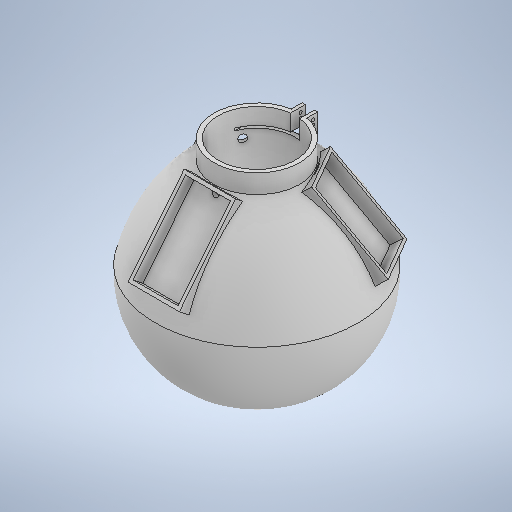
# Autodesk Inventor part: Water Sensor Bouy
Saved by Autodesk Inventor 2025 (Build 290162000, 162)
## iProperties
Created: 2024-06-17
Part Number: Water Sensor Bouy
Material: Generic
Document SubType Name: Modeling
Designer: track
Density: 1 g/cm^3
Appearance: Default
Mass: 1114.84 g
Surface Area: 2537.18 cm^2
Volume: 1114.84 cm^3
Author: track
## iProperties of the stored document Water Sensor Bouy_3DPrint.ipt
Created: 2024-06-17
Part Number: Water Sensor Bouy_3DPrint
Material: Generic
Document SubType Name: Modeling
Designer: track
Density: 1 g/cm^3
Appearance: Default
Author: track
Autodesk Inventor part; units mm, degrees
ref_plane "YZ Plane" through (0, 0, 0) normal (1, 0, 0) x (0, 1, 0)
ref_plane "XZ Plane" through (0, 0, 0) normal (0, 1, 0) x (-1, 0, 0)
ref_plane "XY Plane" through (0, 0, 0) normal (0, 0, 1) x (1, 0, 0)
sketch "Sketch1" plane through (0, 0, 0) normal (0, 0, 1) x (1, 0, 0)
  line L0 (0, 0) -> (0, 76.2)
  line L1 (31.2895, 0) -> (31.2895, 152.4)
  line L2 (31.2895, 76.2) -> (82.0895, 76.2)
  arc A0 (82.0895, 76.2) -> (31.2895, 152.4) centre (-41.8733, 48.5915) ccw
  arc A1 (31.2895, 0) -> (82.0895, 76.2) centre (6.0118, 71.8852) ccw
  line L3 (41.2895, 130.8894) -> (41.2895, 15.868)
  arc A2 (41.2895, 15.868) -> (72.1461, 74.8322) centre (6.0118, 71.8852) ccw
  arc A3 (72.1461, 74.8322) -> (41.2895, 130.8894) centre (-41.8733, 48.5915) ccw
  point P0 (31.2895, 50.8)
  dimension "d1" = 31.2895
  dimension "d3" = 0
  dimension "d74" = 152.4
  dimension "d75" = 50.8
  dimension "d76" = 76.2
  dimension "d78" = 127
  dimension "d83" = 10
  dimension "d128" = 83.1628
  dimension "d129" = 76.2
  constraints: 8 end point, 8 point on circle, 4 centre point, 2 vertical, 1 horizontal, 1 midpoint, 1 point on line, 2 other
  measures "d1" distance between parallel lines of L1 L0
  measures "d3" vertical distance of L0.start L1.start
  measures "d74" distance of L1.start L1.end
  measures "d75" distance of L2.start L2.end
  measures "d76" distance from line of L1.end L2
  measures "d78" radius of A0
  measures "d83" distance between parallel lines of L1 L3
  measures "d128" distance from line of L3 A0.centre
  measures "d129" radius of A1
revolve "Revolution1" add sketch "Sketch1" angle 360 about axis through (0, 0, 0) along (0, 1, 0) contours L1 L2 L3 A2 A3 A1 | L1 A0 L2 A3 L3
sketch "Sketch13" plane through (0, 0, 0) normal (0, 0, 1) x (1, 0, 0)
  line L0 (31.2895, 152.4) -> (-31.2895, 152.4) projected
  line L1 (0, 152.4) -> (0, 180.8136)
  line L2 (-31.2895, 152.4) -> (-31.2895, 165.1)
  line L3 (-31.2895, 165.1) -> (-33.8295, 165.1)
  line L4 (-33.8295, 165.1) -> (-33.8295, 150.5625)
  arc A0 (-31.2895, 152.4) -> (-82.0895, 76.2) centre (41.8733, 48.5915) ccw projected
  arc A1 (-31.2895, 152.4) -> (-33.8295, 150.5625) centre (41.8733, 48.5915) ccw
  point P0 (0, 0)
  dimension "d79" = 2.54
  dimension "d81" = 12.7
  constraints: 8 end point, 3 point on circle, 2 perpendicular, 2 vertical, 1 centre point, 1 concentric, 1 midpoint
  measures "d79" distance of L2.end L3.end
  measures "d81" distance of L0.end L2.end
revolve "Revolution2" add sketch "Sketch13" angle 260 about axis through (0, 152.4, 0) along (0, 1, 0) and the other way 90
sketch "Sketch17" plane through (0, 0, 0) normal (0, 0, 1) x (1, 0, 0)
  line L0 (0, 152.4) -> (0, 165.1) projected
  line L1 (0, 165.1) -> (-8.89, 165.1)
  line L2 (-8.89, 165.1) -> (-8.89, 150.5625)
  line L3 (-8.89, 150.5625) -> (0, 150.5625)
  line L4 (0, 150.5625) -> (0, 165.1)
  point P0 (0, 0)
  dimension "d91" = 8.89
  dimension "d92" = 14.5375
  constraints: 8 end point, 2 parallel, 1 horizontal, 1 perpendicular
  measures "d91" distance of L0.end L1.end
  measures "d92" distance of L1.end L2.end
extrude "Extrusion10" add sketch "Sketch17" along normal blind 2.54
sketch "Sketch18" plane through (0, 152.4, -31.2895) normal (1, 0, 0) x (0, 0, -1)
  line L0 (0, 12.7) -> (2.54, 12.7) projected
  line L1 (0, 0) -> (0, 12.7) projected
  arc A0 (2.54, -1.8375) -> (0, 0) centre (-73.1628, -103.8085) ccw projected
  line L2 (0, 0) -> (-0.4754, 0) projected
  arc A1 (50.8, -76.2) -> (0, 0) centre (-73.1628, -103.8085) ccw projected
  line L3 (0, 0) -> (2.54, -1.8375)
  line L4 (-31.2895, -1.8375) -> (2.54, -1.8375) projected
  line L5 (-33.8295, 12.7) -> (-33.8295, -1.8375) projected
  line L6 (8.89, -1.8375) -> (8.89, 12.7)
  line L7 (-33.8295, 12.7) -> (0, 12.7)
  line L8 (2.54, 12.7) -> (2.54, -1.8375) projected
  point P0 (-31.2895, -152.4)
  constraints: 6 end point, 1 perpendicular, 1 vertical
extrude "Extrusion11" add sketch "Sketch18" along normal blind 12.7 contours L0 L8 A0 L1
sketch "Sketch22" plane through (0, 0, 0) normal (1, 0, 0) x (0, 1, 0)
  arc A0 (150.5625, 33.8295) -> (76.2, 82.0895) centre (48.5915, -41.8733) ccw projected
  arc A1 (76.2, 82.0895) -> (0, 31.2895) centre (71.8852, 6.0118) ccw projected
  line L0 (128.1112, 57.15) -> (74.8322, 12.4436)
  line L1 (74.8322, -72.1461) -> (74.8322, 72.1461) projected
  line L2 (152.4, -31.2895) -> (165.1, -31.2895) projected
  line L3 (74.8322, 0) -> (165.1, 0)
  point P0 (0, 0)
  point P1 (74.8322, 0)
  point P2 (150.5625, 0)
  dimension "d125" = 50
  constraints: 4 end point, 1 horizontal, 1 midpoint, 1 point on circle, 1 point on line, 1 other
  measures "d125" angle of L1 L0
ref_plane "Work Plane6" through (0, 128.1112, 57.15) normal (0, 0.6261398, 0.7797108) x (-1, 0, 0)
sketch "Sketch23" plane through (0, 128.1112, 57.15) normal (0, 0.6261398, 0.7797108) x (-1, 0, 0)
  line L0 (18.25, -27.8894) -> (-18.25, -27.8894)
  line L1 (-18.25, -27.8894) -> (-18.25, 39.6106)
  line L2 (-18.25, 39.6106) -> (18.25, 39.6106)
  line L3 (18.25, 39.6106) -> (18.25, -27.8894)
  ellipse E0 centre (0, -53.2894) end of major axis (-33.8295, -53.2894) minor radius 21.182 (0, -74.4714) -> (-5.8744, -74.1496) ccw projected
  line L4 (-20.79, 42.1506) -> (-20.79, -30.4294)
  line L5 (-20.79, -30.4294) -> (20.79, -30.4294)
  line L6 (20.79, -30.4294) -> (20.79, 42.1506)
  line L7 (20.79, 42.1506) -> (-20.79, 42.1506)
  point P0 (0, 64.1058)
  point P1 (32.2678, -59.651)
  point P2 (33.734, -51.699)
  dimension "d130" = 36.5
  dimension "d131" = 67.5
  dimension "d132" = 25.4
  dimension "d133" = 18.25
  dimension "d134" = 2.54
  constraints: 16 end point, 4 parallel, 2 perpendicular, 1 horizontal, 4 other
  measures "d130" distance of L0.start L0.end
  measures "d131" distance of L0.end L1.end
  measures "d132" distance from line of point (0, -53.289) L0
  measures "d133" distance from line of point (0, -53.289) L1
  measures "d134" distance between parallel lines of L1 L4
extrude "Extrusion14" add sketch "Sketch23" against normal up to surface
sketch "Sketch24" plane through (0, 128.1112, 57.15) normal (0, 0.6261398, 0.7797108) x (-1, 0, 0)
  line L0 (18.25, -27.8894) -> (-18.25, -27.8894) projected
  line L1 (-18.25, -27.8894) -> (-18.25, 39.6106) projected
  line L2 (18.25, -27.8894) -> (-18.25, -27.8894)
  line L3 (-18.25, -27.8894) -> (-18.25, 39.6106)
  line L4 (-18.25, 39.6106) -> (18.25, 39.6106)
  line L5 (18.25, 39.6106) -> (18.25, -27.8894)
  point P0 (0, 64.1058)
  constraints: 8 end point, 2 parallel, 1 horizontal, 1 perpendicular
extrude "Extrusion15" cut sketch "Sketch24" against normal blind 10
sketch "Sketch25" plane through (0, 0, 0) normal (0, 0, 1) x (1, 0, 0)
  circle A0 centre (0, 143.5069) radius 3
  line L0 (-18.25, 149.8569) -> (18.25, 149.8569) projected
  line L1 (18.25, 149.8569) -> (18.25, 97.2264) projected
  point P0 (0, 0)
  dimension "d139" = 6
  dimension "d140" = 6.35
  dimension "d141" = 18.25
  constraints: 1 centre point
  measures "d139" diameter of A0
  measures "d140" distance from line of L0 A0.centre
  measures "d141" distance from line of L1 A0.centre
extrude "Extrusion16" cut sketch "Sketch25" along normal blind 63.5
sketch "Sketch26" plane through (0, 121.8498, 49.3529) normal (0, 0.6261398, 0.7797108) x (1, 0, 0)
  line L0 (-18.25, -39.6106) -> (-18.25, 27.8894) projected
  line L1 (18.25, 27.8894) -> (18.25, -39.6106) projected
  line L2 (-18.25, -14.2106) -> (18.25, -14.2106)
  line L3 (18.25, -14.2106) -> (18.25, -39.6106)
  line L4 (18.25, -39.6106) -> (-18.25, -39.6106)
  line L5 (-18.25, -39.6106) -> (-18.25, -14.2106)
  point P0 (0, -64.1058)
  point P1 (18.25, -14.2106)
  dimension "d144" = 25.4
  constraints: 8 end point, 2 parallel, 1 horizontal, 1 perpendicular, 1 point on line
  measures "d144" distance between parallel lines of L4 L2
extrude "Extrusion17" add sketch "Sketch26" against normal blind 10
pattern_circular "Circular Pattern4" count 3 over 360 about axis through (0, 157.8313, 0) along (0, 1, 0) of "Extrusion14", "Extrusion15", "Extrusion16", "Extrusion17"
sketch "Sketch27" plane through (0, 0, 0) normal (0, 1, 0) x (-1, 0, 0)
  line L0 (0, 0) -> (-82.0895, 0)
  circle A0 centre (0, 0) radius 82.0895 projected
  circle A1 centre (-50.8, 0) radius 3.175
  dimension "d150" = 6.35
  dimension "d151" = 50.8
  constraints: 2 end point, 1 centre point, 1 horizontal, 1 horizontal alignment, 1 point on line, 1 other
  measures "d150" diameter of A1
  measures "d151" distance of L0.start A1.centre
extrude "Extrusion18" cut sketch "Sketch27" along normal blind 33.02 contours A1 L0 | L0 A1
pattern_circular "Circular Pattern5" count 3 over 360 about axis through (0, 71.8852, 0) along (0, 1, 0) of "Extrusion18"
sketch "Sketch30" plane through (0, 165.1, -33.8295) normal (0, 1, 0) x (1, 0, 0)
  line L0 (0, -33.8295) -> (0, -36.3695) projected
  line L1 (12.7, 0) -> (12.7, -2.4744) projected
  circle A0 centre (0, -33.8295) radius 36.1348
  constraints: 1 coincident, 3 other
extrude "Extrusion20" cut sketch "Sketch30" against normal blind 15.24
sketch "Sketch31" plane through (0, 149.86, 0) normal (0, 1, 0) x (1, 0, 0)
  circle A0 centre (0, 0) radius 31.2895
  circle A1 centre (0, 0) radius 31.2895 projected
  circle A2 centre (0, 0) radius 34.7667 projected
  line L0 (6.35, 34.1819) -> (6.35, 43.0719)
  line L1 (6.35, 43.0719) -> (3.81, 43.0719)
  line L2 (3.81, 43.0719) -> (3.81, 34.5573)
  line L3 (-3.81, 34.5573) -> (-3.81, 43.0719)
  line L4 (-3.81, 43.0719) -> (-6.35, 43.0719)
  line L5 (-6.35, 43.0719) -> (-6.35, 34.1819)
  arc A3 (-6.35, 34.1819) -> (6.35, 34.1819) centre (0, 0) ccw
  line L6 (3.81, 34.5573) -> (3.81, 31.0567)
  line L7 (-3.81, 34.5573) -> (-3.81, 31.0567)
  dimension "d165" = 8.89
  dimension "d167" = 8.89
  dimension "d168" = 2.54
  dimension "d169" = 2.54
  dimension "d170" = 3.81
  constraints: 16 end point, 8 point on circle, 3 perpendicular, 2 centre point, 2 coincident, 2 parallel, 2 point on line, 2 vertical, 1 concentric
  measures "d165" distance of L0.start L0.end
  measures "d167" distance of L4.end L5.end
  measures "d168" distance of L3.end L4.end
  measures "d169" distance of L0.end L1.end
  measures "d170" distance from line of point (0, 0) L2
extrude "Extrusion21" add sketch "Sketch31" along normal blind 15.24 contours A0 L6 A2 L7 | L2 L1 L0 A2 | A2 L5 L4 L3 picked at (33.28, -2.7362)
sketch "Sketch32" plane through (-6.35, 149.86, -43.0719) normal (-1, 0, 0) x (0, 0, 1)
  line L0 (0, 15.24) -> (8.89, 15.24) projected
  line L1 (3.81, 15.24) -> (3.81, 0)
  line L2 (0, 0) -> (8.5146, 0) projected
  line L3 (0, 0) -> (0, 15.24) projected
  circle A0 centre (3.81, 11.43) radius 1.27
  circle A1 centre (3.81, 7.62) radius 1.27
  circle A2 centre (3.81, 3.81) radius 1.27
  point P0 (43.0719, -149.86)
  dimension "d173" = 3.81
  dimension "d174" = 2.54
  dimension "d175" = 7.62
  dimension "d176" = 3.81
  dimension "d177" = 3.81
  constraints: 4 point on line, 3 centre point, 2 end point, 2 equal radius, 1 midpoint, 1 vertical
  measures "d173" distance between parallel lines of L3 L1
  measures "d174" diameter of A1
  measures "d175" distance from line of L0 A1.centre
  measures "d176" distance of A1.centre A0.centre
  measures "d177" distance of A1.centre A2.centre
extrude "Extrusion22" cut sketch "Sketch32" against normal up to surface (12.7 mm away) contours A0 L1 | L1 A0 | A2 L1 | L1 A2 | A1 L1 | L1 A1
sketch "Sketch35" plane through (0, 0, 0) normal (0, 0, 1) x (1, 0, 0)
  line L0 (-3.81, 149.86) -> (-6.35, 149.86) projected
  line L1 (-3.81, 149.86) -> (-29.21, 149.86)
  line L2 (-29.21, 149.86) -> (-29.21, 151.765)
  line L3 (-29.21, 151.765) -> (-3.81, 151.765)
  line L4 (-3.81, 151.765) -> (-3.81, 149.86)
  point P0 (0, 0)
  dimension "d181" = 1.905
  dimension "d182" = 25.4
  constraints: 8 end point, 2 parallel, 1 horizontal, 1 perpendicular
  measures "d181" distance of L3.end L0.start
  measures "d182" distance of L2.end L3.end
extrude "Extrusion23" cut sketch "Sketch35" against normal up to surface round surface about axis through (0, 149.86, 0) along (0, 1, 0) radius 34.7667 far side no
sketch "Sketch38" plane through (-3.81, 149.86, -43.0719) normal (0, 0, -1) x (-1, 0, 0)
  line L0 (0, 0) -> (2.54, 0) projected
  line L1 (2.54, 0) -> (2.54, 1.905) projected
  line L2 (0, 0) -> (2.54, 0)
  line L3 (2.54, 0) -> (2.54, 1.905)
  line L4 (2.54, 1.905) -> (0, 1.905)
  line L5 (0, 1.905) -> (0, 0)
  point P0 (-3.81, -149.86)
  constraints: 8 end point, 2 parallel, 1 horizontal, 1 perpendicular
extrude "Extrusion24" cut sketch "Sketch38" against normal blind 25.4
body "Solid1"
